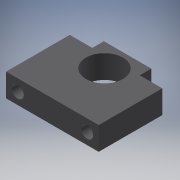
# Autodesk Inventor part: BF 15 Part1
Saved by Autodesk Inventor 2018 (Build 220112000, 112)
## iProperties
Category: PARTsolutions
Company: THK
Created: 2017-05-30
Part Number: BF 15 Part1
Catalog Web Link: www.cadenas.de
Description: Supported side type BF-Part1-
Vendor: THK
Document SubType Name: Modeling
Designer: psAdmin
Manufacturer: THK
Mass: 41.5867 g
Surface Area: 127.439 cm^2
Volume: 41.5867 cm^3
Density: 1 g/cm^3
Material: Generic
Appearance: PSOLRGB-192-192-192
PSOL_IDENT_0: {$CADENAS_DATA\23d-libs\thk\fed_screw\ball_screw\ball_screw_peripheral\suport_unit\supported_bf_1.pr
PSOL_IDENT_1: j},186 {VTYP=3D},{NB=BF 15 Part1},{LINA=BF 15 Part1},{NN=Supported side type BF-Part1},{DATE=16.05.2
PSOL_IDENT_2: 017 06:09:50},{GEOMDATE=08.02.2016 08:57:00},{VERSION=},{LINEID=30},{LINESUBID=-1},{WBVAR=}  {NB=BF
PSOL_IDENT_3: 15 Part1},{LINA=BF 15 Part1},{KT=DUMMY},{IDNR=},{MN=BF 15},{SD=15.000},{L=20.000},{B=70.000},{H=48.0
PSOL_IDENT_4: 00},{SB=35.000},{SH1=28.000},{B1=40.000},{H1=38.000},{E=18.000},{SD3=5.500},{P=54.000},{SD1=6.600},{
PSOL_IDENT_5: SD2=11.000},{SH=6.500},{DK=30.000},{L4=3.500},{SD4=20.000},{D=28.000},{DD=25.000},{P1=1.500},{B2=38.
PSOL_IDENT_6: 000},{D1=7.800},{DX=32.000}
NN: Supported side type BF-Part1
NB: BF 15 Part1
NBSYN: $MN. Part1
LINA: BF 15 Part1
MN: BF 15
SD: 15.000
L: 20.000
B: 70.000
H: 48.000
SB: 35.000
SH1: 28.000
B1: 40.000
H1: 38.000
E: 18.000
SD3: 5.500
P: 54.000
SD1: 6.600
SD2: 11.000
SH: 6.500
DK: 30.000
L4: 3.500
SD4: 20.000
D: 28.000
DD: 25.000
P1: 1.500
B2: 38.000
D1: 7.800
DX: 32.000
SUPPLIER: THK
ARTICLENO: BF 15 Part1
BOMINFO: BF 15 Part1
CREATOR: CADENAS GmbH
Title: BF 15 Part1
Author: Cadenas PARTsolutions
Autodesk Inventor part; units mm, degrees
ref_plane "YZ Plane" through (0, 0, 0) normal (1, 0, 0) x (0, 1, 0)
ref_plane "XZ Plane" through (0, 0, 0) normal (0, 1, 0) x (-1, 0, 0)
ref_plane "XY Plane" through (0, 0, 0) normal (0, 0, 1) x (1, 0, 0)
sketch "Sketch_1" plane through (0, 0, 0) normal (0, 0, 1) x (1, 0, 0)
  line L0 (-40, -45) -> (-40, 10)
  line L1 (-40, 10) -> (-20.5, 10)
  line L2 (-20.5, 10) -> (-20.5, 20)
  line L3 (-20.5, 20) -> (20.5, 20)
  line L4 (20.5, 20) -> (20.5, 10)
  line L5 (20.5, 10) -> (40, 10)
  line L6 (40, 10) -> (40, -45)
  line L7 (40, -45) -> (-40, -45)
  line L8 (-40, -45) -> (-40, -25)
  dimension "d24" = 55
  dimension "d25" = 19.5
  dimension "d26" = 10
  dimension "d27" = 41
  dimension "d28" = 10
  dimension "d29" = 19.5
  dimension "d30" = 55
  dimension "d31" = 20
  constraints: 18 end point, 4 perpendicular, 3 point on line, 1 vertical
  measures "d24" distance of L0.start L0.end
  measures "d25" distance of L0.end L1.end
  measures "d26" distance of L1.end L2.end
  measures "d27" distance of L2.end L3.end
  measures "d28" distance of L3.end L4.end
  measures "d29" distance of L4.end L5.end
  measures "d30" distance of L5.end L6.end
  measures "d31" distance of L0.start L8.end
extrude "Extrusion1" add sketch "Sketch_1" against normal blind 20
ref_plane "bf_1_XY" through (0, 0, 0) normal (0, 0, 1) x (1, 0, 0)
ref_plane "bf_1_YZ" through (0, 0, 0) normal (1, 0, 0) x (0, 1, 0)
ref_plane "bf_1_ZX" through (0, 0, 0) normal (0, 1, 0) x (0, 0, 1)
ref_plane "bf_2x_XY" through (0, 0, -10) normal (0, 0, 1) x (1, 0, 0)
ref_plane "bf_2x_YZ" through (0, 0, -10) normal (1, 0, 0) x (0, 1, 0)
ref_plane "bf_2x_ZX" through (0, 0, -10) normal (0, 1, 0) x (0, 0, 1)
sketch "Sketch7" plane through (0, 0, 0) normal (0, 0, 1) x (1, 0, 0)
  circle A0 centre (0, 0) radius 16
  dimension "d42" = 32
  constraints: 1 centre point, 1 coincident
  measures "d42" diameter of A0
extrude "Extrusion2" cut sketch "Sketch7" against normal up to surface (20 mm away)
sketch "Sketch6" plane through (20.5, 10, 0) normal (0, 1, 0) x (1, 0, 0)
  line L0 (-41, 0) -> (0, 0) projected
  line L1 (19.5, 0) -> (19.5, 20) projected
  line L2 (19.5, 10) -> (9.5, 10)
  line L3 (-60.5, 0) -> (-60.5, 20) projected
  line L4 (-60.5, 10) -> (-50.5, 10)
  point P0 (-20.5, 0)
  dimension "d32" = 10
  dimension "d40" = 10
  constraints: 4 end point, 2 horizontal, 2 midpoint
  measures "d32" distance of L2.start L2.end
  measures "d40" distance of L4.start L4.end
hole "Hole4" at (30, 10, -10) at (-30, 10, -10) direction (0, -1, 0) diameter 10.5 end through all counterbore diameter 17 counterbore depth 12
body "Solid1"
